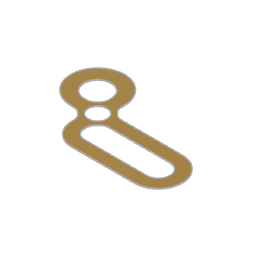
_Test loop.d04cfcd0-42f6-463c-ae4d-885bbe8061d5 (Autodesk Fusion 360 design; units mm, degrees)
Autodesk Fusion 360 part; units mm, degrees
sketch "Sketch1" plane through (0, 0, 0) normal (0, 0, 1) x (1, 0, 0)
sketch "Sketch2" plane through (0, 0, 0) normal (0, 0, 1) x (1, 0, 0)
  circle A0 centre (0, 0) radius 457.2
  circle A1 centre (0, 0) radius 685.8
  line L0 (1018.2819, 304.8) -> (-1018.2819, 304.8)
  line L1 (-1018.2819, 304.8) -> (-1018.2819, -304.8)
  line L2 (-1018.2819, -304.8) -> (1018.2819, -304.8)
  line L3 (1018.2819, -304.8) -> (1018.2819, 304.8)
  line L4 (1018.2819, 304.8) -> (-1018.2819, -304.8) construction
  line L5 (-1018.2819, 304.8) -> (1018.2819, -304.8) construction
  line L6 (304.8, 962.5861) -> (-304.8, 962.5861)
  line L7 (-304.8, 962.5861) -> (-304.8, -962.5861)
  line L8 (-304.8, -962.5861) -> (304.8, -962.5861)
  line L9 (304.8, -962.5861) -> (304.8, 962.5861)
  line L10 (304.8, 962.5861) -> (-304.8, -962.5861) construction
  line L11 (-304.8, 962.5861) -> (304.8, -962.5861) construction
  line L12 (1018.2819, 304.8) -> (3809.9783, 304.8)
  line L13 (3809.9783, 304.8) -> (3809.9783, -304.8)
  line L14 (3809.9783, -304.8) -> (1018.2819, -304.8)
  line L15 (1018.2819, -304.8) -> (1018.2819, 304.8)
  line L16 (304.8, -962.5861) -> (762, -962.5861)
  line L17 (762, -962.5861) -> (762, -1419.7861)
  line L18 (762, -1419.7861) -> (3815.2722, -1419.7861)
  line L19 (3815.2722, -1419.7861) -> (3815.2722, -2029.3861)
  line L20 (3815.2722, -2029.3861) -> (762, -2029.3861)
  line L21 (762, -2029.3861) -> (762, -1419.7861)
  arc A2 (304.8, -962.5861) -> (762, -1419.7861) centre (762, -962.5861) ccw
  arc A3 (-304.8, -962.5861) -> (762, -2029.3861) centre (762, -962.5861) ccw
  arc A4 (3815.2722, -1419.7861) -> (3809.9783, -304.8) centre (3815.2722, -862.2805) ccw
  arc A5 (3815.2722, -2029.3861) -> (3809.9783, 304.8) centre (3815.2722, -862.287) ccw
  circle A6 centre (-999.1399, 999.5225) radius 1304.463
  circle A7 centre (-964.7599, 962.5861) radius 659.9599
  dimension "d1" = 914.4
  dimension "d2" = 1371.6
  dimension "d3" = 609.6
  dimension "d4" = 609.6
  dimension "d5" = 457.2
  dimension "d6" = 457.2
  dimension "d7" = 609.6
  constraint coincident A0.centre A1.centre
  constraint horizontal L0
  constraint perpendicular L0 L1
  constraint parallel L0 L2
  constraint parallel L1 L3
  constraint coincident L4 A0.centre
  constraint coincident L5 A0.centre
  constraint horizontal L6
  constraint perpendicular L6 L7
  constraint parallel L6 L8
  constraint parallel L7 L9
  constraint coincident L10 A0.centre
  constraint coincident L11 A0.centre
  constraint horizontal L12
  constraint vertical L13
  constraint horizontal L14
  constraint vertical L15
  constraint perpendicular L9 L16
  constraint perpendicular L16 L17
  constraint horizontal L18
  constraint vertical L19
  constraint horizontal L20
  constraint vertical L21
  constraint tangent L18 A2
  constraint tangent L20 A3
  constraint tangent L18 A4
  constraint tangent L20 A5
  constraint coincident L1.end A6
  constraint coincident L6.start A6
  constraint coincident L0.end A7
  constraint coincident L6.end A7
  constraint tangent L7 A7
  measures "d1" diameter of A0
  measures "d2" diameter of A1
  measures "d3" distance of L0.end L1.end
  measures "d4" distance of L7.end L8.end
  measures "d5" distance of L8.end L16.end
  measures "d6" distance of L16.end L17.end
  measures "d7" distance of L17.end L20.end
extrude "Extrude1" add sketch "Sketch2" along normal blind 25.4 contours A0 A1 L0 L2 | A0 A1 L0 L9 | A0 A1 L2 L9 | A0 A1 L9 A6 | A1 L0 L2 L3 L15 | A0 A1 L7 L9 | A0 A1 L7 A6 | L3 L12 L13 L14 L15 | A0 A1 L2 L7 | A1 L7 L8 L9 | A0 A1 L0 L7 | A1 L6 L7 A6 | L1 L6 A6 A7 | L13 L19 A4 A5 | A0 A1 L2 A6 | L8 L21 A2 A3 | A0 A1 L0 A6 | L18 L19 L20 L21 | A1 L2 A6 | A1 L0 L1 L2 A6 A7
fillet "Fillet1" radius 457.2 8 edges at (614.344, -304.8, 12.7) (304.8, -614.344, 12.7) (-304.8, -614.344, 12.7) (-614.344, -304.8, 12.7) (-614.344, 304.8, 12.7) (-304.8, 614.344, 12.7) (253.9507, 637.0484, 12.7) (614.344, 304.8, 12.7)
